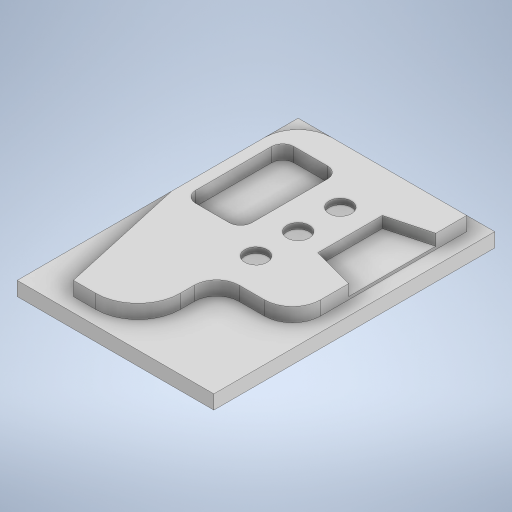
# Autodesk Inventor part: A2P4
Saved by Autodesk Inventor 2023.2 (Build 272271000, 271)
## iProperties
Created: 2023-01-23
Part Number: A2P4
Material: Generic
Document SubType Name: Modeling
Designer: manas
Density: 1 g/cm^3
Appearance: Default
Author: manas
Autodesk Inventor part; units mm, degrees
ref_plane "YZ Plane" through (0, 0, 0) normal (1, 0, 0) x (0, 1, 0)
ref_plane "XZ Plane" through (0, 0, 0) normal (0, 1, 0) x (-1, 0, 0)
ref_plane "XY Plane" through (0, 0, 0) normal (0, 0, 1) x (1, 0, 0)
sketch "Sketch1" plane through (0, 0, 0) normal (0, 1, 0) x (-1, 0, 0)
  line L0 (35, 50) -> (-35, 50)
  line L1 (-35, 50) -> (-35, -50)
  line L2 (-35, -50) -> (35, -50)
  line L3 (35, -50) -> (35, 50)
  line L4 (35, 50) -> (-35, -50) construction
  line L5 (-35, 50) -> (35, -50) construction
  point P0 (0, 0)
  dimension "d0" = 70
  dimension "d1" = 100
  constraints: 12 end point, 2 midpoint, 2 parallel, 1 horizontal, 1 perpendicular
  measures "d0" distance of L2.end L1.end
  measures "d1" distance of L1.end L0.end
extrude "Extrusion1" add sketch "Sketch1" along normal blind 5
sketch "Sketch2" plane through (0, 5, 0) normal (0, 1, 0) x (1, 0, 0)
  line L0 (-20, -45) -> (-12, -45)
  line L1 (30, -7) -> (30, 45)
  line L2 (30, 45) -> (-18, 45)
  line L3 (-30, 33) -> (-30, 0)
  line L4 (-30, -45) -> (30, 45) construction
  line L5 (30, -45) -> (-30, 45) construction
  line L6 (-20, -45) -> (-30, 0)
  line L7 (-35, -50) -> (35, -50) projected
  line L8 (35, -50) -> (35, 50) projected
  line L9 (3, -25) -> (3, -30)
  line L10 (20, -17) -> (11, -17)
  arc A0 (11, -17) -> (3, -25) centre (11, -25) ccw
  arc A1 (20, -17) -> (30, -7) centre (20, -7) ccw
  arc A2 (-18, 45) -> (-30, 33) centre (-18, 33) ccw
  line L11 (-22, 0.5) -> (-10, 0.5)
  line L12 (-6, 4.5) -> (-6, 31.5)
  line L13 (-10, 35.5) -> (-22, 35.5)
  line L14 (-26, 31.5) -> (-26, 4.5)
  line L15 (-26, 0.5) -> (-6, 35.5) construction
  line L16 (-6, 0.5) -> (-26, 35.5) construction
  arc A3 (-12, -45) -> (3, -30) centre (-12, -30) ccw
  arc A4 (-26, 4.5) -> (-22, 0.5) centre (-22, 4.5) ccw
  arc A5 (-22, 35.5) -> (-26, 31.5) centre (-22, 31.5) ccw
  arc A6 (-6, 31.5) -> (-10, 35.5) centre (-10, 31.5) ccw
  arc A7 (-10, 0.5) -> (-6, 4.5) centre (-10, 4.5) ccw
  point P0 (0, 0)
  point P1 (3, -45)
  point P2 (-16, 18)
  dimension "d4" = 60
  dimension "d5" = 90
  dimension "d6" = 50
  dimension "d7" = 55
  dimension "d8" = 32
  dimension "d10" = 8
  dimension "d11" = 10
  dimension "d12" = 12
  dimension "d22" = 20
  dimension "d23" = 35
  dimension "d24" = 68
  dimension "d25" = 51
  dimension "d26" = 15
  dimension "d39" = 4
  constraints: 30 end point, 16 point on circle, 16 tangent, 12 point on line, 8 centre point, 4 midpoint, 4 parallel, 3 equal radius, 3 horizontal, 3 perpendicular
  measures "d4" distance of L5.end L1.end
  measures "d5" distance of L1.end L5.start
  measures "d6" distance from line of L3.end L7
  measures "d7" distance from line of L0.start L8
  measures "d8" distance between parallel lines of L8 L9
  measures "d10" radius of A0
  measures "d11" radius of A1
  measures "d12" radius of A2
  measures "d22" distance of L16.end L15.end
  measures "d23" distance of L15.end L16.start
  measures "d24" distance from line of L7 point (-16, 18)
  measures "d25" distance from line of L8 point (-16, 18)
  measures "d26" radius of A3
  measures "d39" radius of A4
extrude "Extrusion2" add sketch "Sketch2" along normal blind 5
sketch "Sketch3" plane through (0, 10, 0) normal (0, 1, 0) x (1, 0, 0)
  line L0 (15, 7) -> (15, 30)
  line L1 (15, 30) -> (30, 34)
  line L2 (30, -7) -> (30, 45) projected
  line L3 (15, 7) -> (30, 3)
  line L4 (-35, -50) -> (35, -50) projected
  line L5 (30, 3) -> (30, 34)
  point P0 (0, 0)
  dimension "d15" = 23
  dimension "d16" = 15
  dimension "d17" = 53
  dimension "d18" = 57
  dimension "d19" = 84
  constraints: 8 end point, 2 point on line, 1 collinear, 1 vertical
  measures "d15" distance of L0.start L0.end
  measures "d16" distance between parallel lines of L2 L0
  measures "d17" distance from line of L4 L3.end
  measures "d18" distance from line of L4 L0.start
  measures "d19" distance from line of L4 L1.end
extrude "Extrusion3" cut sketch "Sketch3" against normal blind 4
sketch "Sketch4" plane through (0, 10, 0) normal (0, 1, 0) x (1, 0, 0)
  circle A0 centre (5, -5) radius 4
  line L0 (-35, -50) -> (35, -50) projected
  line L1 (35, -50) -> (35, 50) projected
  circle A1 centre (5, 10) radius 4
  circle A2 centre (5, 25) radius 4
  point P0 (0, 0)
  dimension "d27" = 8
  dimension "d28" = 45
  dimension "d29" = 30
  dimension "d32" = 15
  constraints: 3 centre point, 1 vertical, 4 other
  measures "d27" diameter of A0
  measures "d28" distance from line of L0 A0.centre
  measures "d29" distance from line of L1 A0.centre
  measures "d32" distance of A0.centre A1.centre
extrude "Extrusion4" cut sketch "Sketch4" against normal blind 2
body "Solid1"
